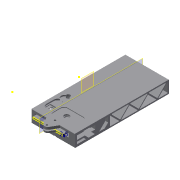
# Autodesk Inventor part: 01_SARS_detector_transmission_H20P_base_v0
Saved by Autodesk Inventor 2019.4 (Build 234330000, 330)
## iProperties
Created: 2020-10-16
Part Number: 01_SARS_detector_transmission_H20P_base_v0
Material: Generic
Document SubType Name: Modeling
Designer: diederichbenedict
Density: 1 g/cm^3
Appearance: Default
Author: diederichbenedict
Autodesk Inventor part; units mm, degrees
(part 1 of 2)
ref_plane "XZ Plane" through (0, 0, 0) normal (0, 1, 0) x (-1, 0, 0)
ref_plane "Work Plane1" through (47, 0, 0) normal (1, 0, 0) x (0, 1, 0)
sketch "Sketch1" plane through (47, 0, 0) normal (1, 0, 0) x (0, 1, 0)
  line L0 (-12.299, 54.1973) -> (-12.299, -85.8027) projected
  line L1 (-7.299, 21.1973) -> (-12.299, 21.1973)
  line L2 (-7.299, 17.1973) -> (-12.299, 17.1973)
  line L3 (-12.299, 21.6973) -> (-19.299, 21.6973)
  line L4 (-24.299, 26.6973) -> (-24.299, 42.4673)
  line L5 (-12.299, 51.1973) -> (-12.299, 56.0473) projected
  line L6 (-12.799, 51.1973) -> (-12.799, 56.0473) projected
  line L7 (-12.299, 54.1973) -> (-12.299, 57.6973) projected
  line L8 (-12.299, 56.3123) -> (-12.299, 70.3123)
  line L9 (-12.299, 56.3123) -> (-15.299, 56.3123)
  line L10 (-15.299, 56.3123) -> (-15.299, 21.6973)
  line L11 (-12.299, 16.6973) -> (-23.299, 16.6973)
  line L12 (-23.299, 16.6973) -> (-28.765, 22.1633)
  line L13 (-28.765, 22.1633) -> (-28.765, 48.2313)
  line L14 (-28.765, 48.2313) -> (-20.684, 56.3123)
  line L15 (-20.684, 56.3123) -> (-15.299, 56.3123)
  line L16 (-24.299, 42.4673) -> (-20.684, 46.0823)
  line L17 (-24.299, 42.4673) -> (-19.1866, 42.4673) construction
  line L18 (-20.684, 46.0823) -> (-15.299, 46.0823)
  line L19 (-19.299, 21.6973) -> (-24.299, 26.6973)
  line L20 (-12.999, 46.3323) -> (-17.739, 46.3323) projected
  line L21 (-17.739, 56.0623) -> (-12.999, 56.0623) projected
  line L22 (-12.299, 21.6973) -> (-12.299, 23.2191)
  line L23 (-15.299, 23.2191) -> (-12.299, 23.2191)
  line L24 (-12.299, 70.3123) -> (-32.299, 70.3123)
  line L25 (-32.299, 70.3123) -> (-32.299, -81.6877)
  line L26 (-32.299, -81.6877) -> (-12.299, -81.6877)
  line L27 (-12.299, -81.6877) -> (-12.299, 16.6973)
  line L28 (-12.299, -81.6877) -> (-32.299, -81.6877) construction
  line L29 (-32.299, -81.6877) -> (-32.299, 16.6973) construction
  line L30 (-32.299, 16.6973) -> (-12.299, 16.6973) construction
  line L31 (-12.299, 16.6973) -> (-12.299, -81.6877) construction
  line L32 (-14.299, -79.6877) -> (-30.299, -79.6877)
  line L33 (-30.299, -79.6877) -> (-30.299, 13.6973)
  line L34 (-30.299, 13.6973) -> (-14.299, 13.6973)
  line L35 (-14.299, 13.6973) -> (-14.299, -79.6877)
  line L36 (-12.299, 16.6973) -> (-15.299, 16.6973)
  line L37 (-15.299, 16.6973) -> (-15.299, 21.6973)
  line L38 (-15.299, 21.6973) -> (-12.299, 21.6973)
  line L39 (-12.299, 21.6973) -> (-12.299, 16.6973)
  line L40 (-12.299, 19.1973) -> (-25.799, 19.1973) construction
  line L41 (-25.799, 51.1973) -> (-12.799, 51.1973) construction
  line L42 (-25.799, 51.1973) -> (-25.799, 19.1973) construction
  line L43 (-28.6297, 52.6092) -> (-25.1023, 56.1367)
  line L44 (-25.1023, 56.1367) -> (-25.1023, 67.0836)
  line L45 (-25.1023, 67.0836) -> (-28.6297, 67.0836)
  line L46 (-28.6297, 67.0836) -> (-28.6297, 52.6092)
  point P0 (0, 0)
  point P1 (-24.299, 21.6973)
  dimension "d4" = 14
  dimension "d6" = 135
  dimension "d7" = 135
  dimension "d8" = 135
  dimension "d9" = 45
  dimension "d10" = 135
  dimension "d11" = 5
  dimension "d13" = 0.25
  dimension "d14" = 0.25
  dimension "d15" = 0.5
  dimension "d16" = 0.5
  dimension "d18" = 0
  dimension "d19" = 12
  dimension "d20" = 20
  dimension "d21" = 152
  dimension "d22" = 90
  dimension "d23" = 2
  dimension "d24" = 2
  dimension "d25" = 2
  dimension "d26" = 3
  dimension "d60" = 13.5
  dimension "d89" = 3
  constraints: 82 end point, 12 horizontal, 11 perpendicular, 9 point on line, 7 parallel, 4 vertical, 1 coincident, 1 collinear, 1 equal length, 1 midpoint, 9 other
  measures "d4" distance of L8.start L8.end
  measures "d6" angle of L11 L12
  measures "d7" angle of L12 L13
  measures "d8" angle of L13 L14
  measures "d9" angle of L17 L16
  measures "d10" angle of L18 L16
  measures "d11" distance of L3.end point (-24.299, 21.697)
  measures "d13" distance between parallel lines of L20 L18
  measures "d14" distance between parallel lines of L15 L21
  measures "d15" distance between parallel lines of L3 L1
  measures "d16" distance between parallel lines of L11 L2
  measures "d18" horizontal distance of L14.end L16.end
  measures "d20" distance of L8.end L24.end
  measures "d21" distance of L24.end L25.end
  measures "d22" angle of L25 L24
  measures "d24" distance between parallel lines of L26 L32
  measures "d25" distance between parallel lines of L29 L33
  measures "d26" distance between parallel lines of L30 L34
  measures "d60" distance of L40.end L40.start
  measures "d89" distance between parallel lines of L14 L43
extrude "Extrusion1" add sketch "Sketch1" along normal blind 50 and the other way blind 20 contours L0 L23 L10 L9 L7 L5 | L0 L3 L10 L23 | L9 L15 L14 L13 L12 L11 L0 L26 L25 L24 L8 L7 | L0 L11 L37 L3 | L10 L3 L19 L4 L16 L18
sketch "Sketch2" plane through (27, 0, 0) normal (-1, 0, 0) x (0, 0, 1)
  line L0 (13.6973, -30.299) -> (-79.6877, -30.299) projected
  line L1 (-79.6877, -30.299) -> (-79.6877, -14.299) projected
  line L2 (-79.6877, -14.299) -> (13.6973, -14.299) projected
  line L3 (13.6973, -14.299) -> (13.6973, -30.299) projected
  line L4 (70.3123, -12.299) -> (-81.6877, -12.299) projected
  line L5 (21.6973, -15.299) -> (21.6973, -19.299) projected
  line L6 (21.6973, -19.299) -> (26.6973, -24.299) projected
  line L7 (26.6973, -24.299) -> (42.4673, -24.299) projected
  line L8 (42.4673, -24.299) -> (46.0823, -20.684) projected
  line L9 (46.0823, -20.684) -> (46.0823, -15.299) projected
  line L10 (46.0823, -15.299) -> (56.3123, -15.299) projected
  line L11 (56.3123, -15.299) -> (56.3123, -20.684) projected
  line L12 (56.3123, -20.684) -> (48.2313, -28.765) projected
  line L13 (48.2313, -28.765) -> (22.1633, -28.765) projected
  line L14 (22.1633, -28.765) -> (16.6973, -23.299) projected
  line L15 (16.6973, -23.299) -> (16.6973, -15.299) projected
  line L16 (-81.6877, -12.299) -> (-81.6877, -32.299) projected
  line L17 (-81.6877, -32.299) -> (70.3123, -32.299) projected
  line L18 (70.3123, -32.299) -> (70.3123, -12.299) projected
  line L19 (-79.6877, -14.299) -> (-63.6877, -30.299)
  line L20 (-79.6877, -14.299) -> (-57.0603, -14.299) construction
  line L21 (-63.6877, -30.299) -> (-62.1877, -30.299)
  line L22 (-62.1877, -30.299) -> (-46.1877, -14.299)
  line L23 (-46.1877, -14.299) -> (-46.1877, -14.299)
  line L24 (-77.5664, -14.299) -> (-62.9377, -28.9277)
  line L25 (-62.9377, -28.9277) -> (-48.309, -14.299)
  line L26 (-79.6877, -14.299) -> (-77.5664, -14.299)
  line L27 (-48.309, -14.299) -> (-46.1877, -14.299)
  line L28 (16.6973, -15.299) -> (21.6973, -15.299) projected
  point P0 (0, 0)
  dimension "d31" = 45
  dimension "d_1" = 1.5
  dimension "d33" = 135
  dimension "d34" = 0
  dimension "d44" = 0.75
  dimension "d46" = 1.5
  constraints: 18 end point, 5 point on line, 2 collinear, 1 equal length, 1 horizontal, 1 parallel, 1 perpendicular
  measures "d31" angle of L19 L20
  measures "d_1" distance of L19.end L21.end
  measures "d33" angle of L22 L21
  measures "d34" distance of L22.end L23.end
  measures "d44" horizontal distance of L24.end L21.end
  measures "d46" distance between parallel lines of L22 L25
extrude "Extrusion2" add sketch "Sketch2" against normal up to surface (70 mm away) contours L0 L19 L2 L24 L25 L22
pattern_linear "Rectangular Pattern1" count 3 spacing 30 along (0, 0, 1) of "Extrusion2"
fillet "Fillet1" radius 0.75 20 edges at (62, -14.299, -79.6877) (62, -14.299, -77.5664) (62, -28.9277, -62.9377) (62, -30.299, -63.6877) (62, -30.299, -62.1877) (62, -16.049, -47.9377) (62, -16.049, -17.9377) (62, -28.9277, -32.9377) (62, -28.9277, -2.9377) (62, -30.299, 13.6973) (62, -30.299, -2.1877) (62, -30.299, -32.1877) (62, -30.299, -33.6877) (62, -30.299, -3.6877) (62, -14.299, 11.691) (62, -30.299, -79.6877) (62, -12.299, -81.6877) (62, -32.299, -81.6877) (62, -12.299, 70.3123) (62, -32.299, 70.3123)
sketch "Sketch3" plane through (27, -12.299, 69.5623) normal (0, 1, 0) x (1, 0, 0)
  line L0 (6.499, 14) -> (6.499, 22.73) projected
  arc A0 (6.999, 23.23) -> (6.499, 22.73) centre (6.999, 22.73) ccw projected
  arc A1 (6.499, 14) -> (6.999, 13.5) centre (6.999, 14) ccw projected
  line L1 (6.499, 14) -> (6.499, 22.73) projected
  line L2 (15.729, 13.5) -> (6.999, 13.5) projected
  arc A2 (15.729, 13.5) -> (16.229, 14) centre (15.729, 14) ccw projected
  line L3 (16.229, 22.73) -> (16.229, 14) projected
  arc A3 (16.229, 22.73) -> (15.729, 23.23) centre (15.729, 22.73) ccw projected
  line L4 (15.729, 23.23) -> (6.999, 23.23) projected
  line L5 (15.364, 14.75) -> (15.364, 22.75)
  line L6 (15.364, 22.75) -> (7.364, 22.75)
  line L7 (7.364, 22.75) -> (7.364, 14.75)
  line L8 (7.364, 14.75) -> (15.364, 14.75)
  circle A4 centre (11.364, 18.75) radius 4
  line L9 (0, -0.75) -> (70, -0.75) projected
  circle A5 centre (11.364, 47.25) radius 3
  point P0 (-27, 69.5623)
  dimension "d112" = 8
  dimension "d113" = 19.5
  dimension "d114" = 0
  dimension "d115" = 6
  dimension "d116" = 48
  constraints: 8 end point, 3 tangent, 2 centre point, 2 parallel, 1 perpendicular
  measures "d112" diameter of A4
  measures "d113" distance from line of A4.centre L9
  measures "d114" distance edge to line of A4 L6
  measures "d115" diameter of A5
  measures "d116" distance from line of L9 A5.centre
ref_plane "Work Plane2" through (7.664, -19.539, 38.4473) normal (0, -1, 0) x (1, 0, 0)
extrude "Extrusion3" cut sketch "Sketch3" against normal blind 10 contours L0 A0 L4 A3 L3 A2 L2 A1 | L8 A4 L5 | A4 L6 L5 | A4 | L8 L7 A4 | A4 L7 L6 | A5
sketch "Sketch4" plane through (27, 0, 0) normal (-1, 0, 0) x (0, 0, 1)
  line L0 (63.9473, -19.539) -> (38.4473, -19.539) construction
  line L1 (63.9473, -19.539) -> (63.9473, -18.239) construction
  line L2 (38.4473, -18.239) -> (63.9473, -18.239) construction
  line L3 (38.4473, -19.539) -> (38.4473, -18.239) construction
  line L4 (33.4473, -16.239) -> (71.8146, -16.239)
  line L5 (71.8146, -16.239) -> (71.8146, -22.539)
  line L6 (71.8146, -22.539) -> (33.4473, -22.539)
  line L7 (33.4473, -22.539) -> (33.4473, -16.239)
  point P0 (0, 0)
  dimension "d61" = 5
  dimension "d63" = 2
  dimension "d64" = 3
  constraints: 8 end point, 2 parallel, 1 horizontal, 1 perpendicular
  measures "d61" distance between parallel lines of L3 L7
  measures "d63" distance between parallel lines of L2 L4
  measures "d64" distance between parallel lines of L0 L6
extrude "Extrusion4" cut sketch "Sketch4" against normal blind 60
sketch "Sketch5" plane through (27, 0, 0) normal (-1, 0, 0) x (0, 0, 1)
  line L0 (33.4473, -16.239) -> (46.0823, -16.239) projected
  line L1 (46.0823, -16.239) -> (46.0823, -15.299) projected
  line L2 (46.0823, -15.299) -> (56.3123, -15.299) projected
  line L3 (56.3123, -15.299) -> (56.3123, -16.239) projected
  line L4 (56.3123, -16.239) -> (70.3123, -16.239) projected
  line L5 (70.3123, -22.539) -> (54.4573, -22.539) projected
  line L6 (54.4573, -22.539) -> (48.2313, -28.765) projected
  line L7 (48.2313, -28.765) -> (22.1633, -28.765) projected
  line L8 (22.1633, -28.765) -> (16.6973, -23.299) projected
  line L9 (16.6973, -23.299) -> (16.6973, -15.299) projected
  line L10 (16.6973, -15.299) -> (21.6973, -15.299) projected
  line L11 (21.6973, -15.299) -> (21.6973, -19.299) projected
  line L12 (21.6973, -19.299) -> (26.6973, -24.299) projected
  line L13 (26.6973, -24.299) -> (42.4673, -24.299) projected
  line L14 (42.4673, -24.299) -> (44.2273, -22.539) projected
  line L15 (44.2273, -22.539) -> (33.4473, -22.539) projected
  line L16 (33.4473, -22.539) -> (33.4473, -16.239) projected
  arc A0 (69.5623, -32.299) -> (70.3123, -31.549) centre (69.5623, -31.549) ccw projected
  line L17 (70.3123, -31.549) -> (70.3123, -22.539) projected
  arc A1 (70.3123, -13.049) -> (69.5623, -12.299) centre (69.5623, -13.049) ccw projected
  line L18 (69.5623, -12.299) -> (-80.9377, -12.299) projected
  arc A2 (-80.9377, -12.299) -> (-81.6877, -13.049) centre (-80.9377, -13.049) ccw projected
  line L19 (-81.6877, -13.049) -> (-81.6877, -31.549) projected
  arc A3 (-81.6877, -31.549) -> (-80.9377, -32.299) centre (-80.9377, -31.549) ccw projected
  line L20 (-80.9377, -32.299) -> (69.5623, -32.299) projected
  line L21 (13.6973, -14.414) -> (13.6973, -29.549) projected
  arc A4 (12.9473, -30.299) -> (13.6973, -29.549) centre (12.9473, -29.549) ccw projected
  line L22 (12.9473, -30.299) -> (-0.377, -30.299) projected
  line L23 (13.6973, -14.414) -> (-0.9074, -29.0187) projected
  line L24 (-4.968, -29.0187) -> (-17.4074, -16.5793) projected
  line L25 (-18.468, -16.5793) -> (-30.9074, -29.0187) projected
  line L26 (-2.4074, -28.3973) -> (10.4107, -15.5793) projected
  arc A5 (-3.468, -28.3973) -> (-2.4074, -28.3973) centre (-2.9377, -27.867) ccw projected
  line L27 (-16.877, -14.9883) -> (-3.468, -28.3973) projected
  line L28 (-16.1877, -14.299) -> (9.8803, -14.299) projected
  arc A6 (10.4107, -15.5793) -> (9.8803, -14.299) centre (9.8803, -15.049) ccw projected
  line L29 (-32.4074, -28.3973) -> (-18.9983, -14.9883) projected
  arc A7 (-33.468, -28.3973) -> (-32.4074, -28.3973) centre (-32.9377, -27.867) ccw projected
  line L30 (-46.877, -14.9883) -> (-33.468, -28.3973) projected
  line L31 (-46.1877, -14.299) -> (-19.6877, -14.299) projected
  line L32 (-34.968, -29.0187) -> (-47.4074, -16.5793) projected
  line L33 (-48.468, -16.5793) -> (-60.9074, -29.0187) projected
  line L34 (-62.4074, -28.3973) -> (-48.9983, -14.9883) projected
  arc A8 (-63.468, -28.3973) -> (-62.4074, -28.3973) centre (-62.9377, -27.867) ccw projected
  line L35 (-76.286, -15.5793) -> (-63.468, -28.3973) projected
  arc A9 (-75.7557, -14.299) -> (-76.286, -15.5793) centre (-75.7557, -15.049) ccw projected
  line L36 (-75.7557, -14.299) -> (-49.6877, -14.299) projected
  line L37 (-64.968, -29.0187) -> (-78.4074, -15.5793) projected
  arc A10 (-79.6877, -29.549) -> (-78.9377, -30.299) centre (-78.9377, -29.549) ccw projected
  line L38 (-79.6877, -29.549) -> (-79.6877, -16.1096) projected
  arc A11 (-78.4074, -15.5793) -> (-79.6877, -16.1096) centre (-78.9377, -16.1096) ccw projected
  line L39 (63.9473, -19.539) -> (38.4473, -19.539) projected
  line L40 (63.9473, -19.539) -> (63.9473, -18.239) projected
  line L41 (38.4473, -18.239) -> (63.9473, -18.239) projected
  line L42 (38.4473, -19.539) -> (38.4473, -18.239) projected
  line L43 (35.4473, -18.239) -> (35.4473, -19.439)
  line L44 (33.4473, -19.439) -> (33.4473, -18.239)
  line L45 (35.4473, -18.239) -> (37.4473, -18.239)
  line L46 (37.4473, -18.239) -> (37.4473, -20.739)
  line L47 (37.4473, -20.739) -> (35.4473, -20.739)
  line L48 (35.4473, -20.739) -> (35.4473, -18.239)
  line L49 (37.4473, -20.739) -> (64.4473, -20.739)
  line L50 (64.4473, -20.739) -> (64.4473, -19.739)
  line L51 (64.4473, -19.739) -> (37.4473, -19.739)
  line L52 (37.4473, -19.739) -> (37.4473, -20.739)
  line L53 (64.4473, -20.739) -> (74.4473, -20.739)
  line L54 (74.4473, -20.739) -> (74.4473, -18.239)
  line L55 (74.4473, -18.239) -> (64.4473, -18.239)
  line L56 (64.4473, -18.239) -> (64.4473, -20.739)
  line L57 (70.3123, -16.239) -> (70.3123, -13.049) projected
  line L58 (67.0836, -25.1023) -> (67.0836, -28.6297) projected
  line L59 (67.0836, -28.6297) -> (52.6092, -28.6297) projected
  line L60 (52.6092, -28.6297) -> (56.1367, -25.1023) projected
  line L61 (56.1367, -25.1023) -> (67.0836, -25.1023) projected
  arc A12 (-17.4074, -16.5793) -> (-18.468, -16.5793) centre (-17.9377, -17.1096) ccw projected
  arc A13 (-47.4074, -16.5793) -> (-48.468, -16.5793) centre (-47.9377, -17.1096) ccw projected
  line L62 (-5.4983, -30.299) -> (-30.377, -30.299) projected
  arc A14 (-30.9074, -29.0187) -> (-30.377, -30.299) centre (-30.377, -29.549) ccw projected
  arc A15 (-5.4983, -30.299) -> (-4.968, -29.0187) centre (-5.4983, -29.549) ccw projected
  arc A16 (-0.9074, -29.0187) -> (-0.377, -30.299) centre (-0.377, -29.549) ccw projected
  line L63 (-16.1877, -14.299) -> (-16.877, -14.9883) projected
  line L64 (-18.9983, -14.9883) -> (-19.6877, -14.299) projected
  line L65 (-46.1877, -14.299) -> (-46.877, -14.9883) projected
  line L66 (-48.9983, -14.9883) -> (-49.6877, -14.299) projected
  line L67 (-35.4983, -30.299) -> (-60.377, -30.299) projected
  arc A17 (-60.9074, -29.0187) -> (-60.377, -30.299) centre (-60.377, -29.549) ccw projected
  arc A18 (-35.4983, -30.299) -> (-34.968, -29.0187) centre (-35.4983, -29.549) ccw projected
  line L68 (-65.4983, -30.299) -> (-78.9377, -30.299) projected
  arc A19 (-65.4983, -30.299) -> (-64.968, -29.0187) centre (-65.4983, -29.549) ccw projected
  line L69 (35.4473, -20.739) -> (33.4473, -20.739)
  line L70 (33.4473, -20.739) -> (33.4473, -19.739)
  line L71 (33.4473, -19.739) -> (35.4473, -19.739)
  line L72 (35.4473, -19.739) -> (35.4473, -20.739)
  point P0 (0, 0)
  dimension "d67" = 2
  dimension "d68" = 1.2
  dimension "d69" = 2
  dimension "d70" = 2.5
  dimension "d71" = 1
  dimension "d72" = 27
  dimension "d73" = 10
  dimension "d98" = 0
  constraints: 36 end point, 9 parallel, 4 horizontal, 4 perpendicular, 2 point on line
  measures "d67" distance of L43.end L44.start
  measures "d68" distance of L43.start L43.end
  measures "d69" distance of L46.end L47.end
  measures "d70" distance of L45.end L46.end
  measures "d71" distance of L50.end L49.end
  measures "d72" distance between parallel lines of L50 L46
  measures "d73" distance of L55.end L54.end
  measures "d98" distance between parallel lines of L45 L41
extrude "Extrusion5" add sketch "Sketch5" against normal blind 55 contours L71 L48 L69 L16 | L48 L43 L45 L46 L47 | L46 L51 L50 L49 | L50 L56 L55 L54 L53
sketch "Sketch6" plane through (27, -12.299, 69.5623) normal (0, 1, 0) x (1, 0, 0)
  circle A0 centre (11.364, 50.365) radius 2 projected
  arc A1 (16.214, 29.865) -> (6.514, 29.865) centre (11.364, 29.865) ccw projected
  line L0 (6.514, 29.865) -> (6.514, 18.365) projected
  arc A2 (6.514, 18.365) -> (16.214, 18.365) centre (11.364, 18.365) ccw projected
  line L1 (16.214, 18.365) -> (16.214, 29.865) projected
  circle A3 centre (11.364, 41.365) radius 4.315 projected
  arc A4 (6.364, 158.865) -> (2.864, 155.365) centre (6.364, 155.365) ccw projected
  line L2 (65.244, 158.865) -> (6.364, 158.865) projected
  arc A5 (68.744, 155.365) -> (65.244, 158.865) centre (65.244, 155.365) ccw projected
  line L3 (68.744, 15.365) -> (68.744, 155.365) projected
  arc A6 (65.244, 11.865) -> (68.744, 15.365) centre (65.244, 15.365) ccw projected
  line L4 (6.364, 11.865) -> (65.244, 11.865) projected
  arc A7 (2.864, 15.365) -> (6.364, 11.865) centre (6.364, 15.365) ccw projected
  line L5 (2.864, 155.365) -> (2.864, 15.365) projected
  arc A8 (17.714, 29.865) -> (5.014, 29.865) centre (11.364, 29.865) ccw
  line L6 (5.014, 29.865) -> (5.014, 18.365)
  arc A9 (5.014, 18.365) -> (17.714, 18.365) centre (11.364, 18.365) ccw
  line L7 (17.714, 18.365) -> (17.714, 29.865)
  circle A10 centre (11.364, 41.365) radius 5.815
  point P0 (-27, 69.5623)
  dimension "d76" = 1.5
  dimension "d77" = 1.5
  constraints: 4 end point, 4 point on circle, 3 centre point, 3 other
  measures "d76" distance between parallel lines of L1 L7
  measures "d77" radial gap between concentric circles of A3 A10
extrude "Extrusion6" cut sketch "Sketch6" against normal blind 2 contours L1 A2 L0 A1 | A3 | L7 A9 L6 A8 A10 | A10 A8 | A8 A10
sketch "Sketch7" plane through (27, 0, 0) normal (-1, 0, 0) x (0, 0, 1)
  line L0 (70.3123, -22.539) -> (54.4573, -22.539) projected
  line L1 (54.4573, -22.539) -> (48.2313, -28.765) projected
  line L2 (48.2313, -28.765) -> (22.1633, -28.765) projected
  line L3 (22.1633, -28.765) -> (16.6973, -23.299) projected
  line L4 (16.6973, -23.299) -> (16.6973, -15.299) projected
  line L5 (16.6973, -15.299) -> (21.6973, -15.299) projected
  line L6 (21.6973, -15.299) -> (21.6973, -19.299) projected
  line L7 (21.6973, -19.299) -> (26.6973, -24.299) projected
  line L8 (26.6973, -24.299) -> (42.4673, -24.299) projected
  line L9 (42.4673, -24.299) -> (44.2273, -22.539) projected
  line L10 (44.2273, -22.539) -> (33.4473, -22.539) projected
  line L11 (33.4473, -22.539) -> (33.4473, -20.739) projected
  line L12 (33.4473, -16.239) -> (46.0823, -16.239) projected
  line L13 (46.0823, -16.239) -> (46.0823, -15.299) projected
  line L14 (46.0823, -15.299) -> (56.3123, -15.299) projected
  line L15 (56.3123, -15.299) -> (56.3123, -16.239) projected
  line L16 (56.3123, -16.239) -> (70.3123, -16.239) projected
  line L17 (70.3123, -16.239) -> (70.3123, -13.049) projected
  arc A0 (70.3123, -13.049) -> (69.5623, -12.299) centre (69.5623, -13.049) ccw projected
  line L18 (69.5623, -12.299) -> (-80.9377, -12.299) projected
  arc A1 (-80.9377, -12.299) -> (-81.6877, -13.049) centre (-80.9377, -13.049) ccw projected
  line L19 (-81.6877, -13.049) -> (-81.6877, -31.549) projected
  arc A2 (-81.6877, -31.549) -> (-80.9377, -32.299) centre (-80.9377, -31.549) ccw projected
  line L20 (-80.9377, -32.299) -> (69.5623, -32.299) projected
  arc A3 (69.5623, -32.299) -> (70.3123, -31.549) centre (69.5623, -31.549) ccw projected
  line L21 (70.3123, -31.549) -> (70.3123, -22.539) projected
  line L22 (-64.968, -29.0187) -> (-78.4074, -15.5793) projected
  line L23 (-65.4983, -30.299) -> (-78.9377, -30.299) projected
  arc A4 (-79.6877, -29.549) -> (-78.9377, -30.299) centre (-78.9377, -29.549) ccw projected
  line L24 (-79.6877, -29.549) -> (-79.6877, -16.1096) projected
  arc A5 (-78.4074, -15.5793) -> (-79.6877, -16.1096) centre (-78.9377, -16.1096) ccw projected
  line L25 (-62.4074, -28.3973) -> (-48.9983, -14.9883) projected
  arc A6 (-63.468, -28.3973) -> (-62.4074, -28.3973) centre (-62.9377, -27.867) ccw projected
  line L26 (-76.286, -15.5793) -> (-63.468, -28.3973) projected
  arc A7 (-75.7557, -14.299) -> (-76.286, -15.5793) centre (-75.7557, -15.049) ccw projected
  line L27 (-75.7557, -14.299) -> (-49.6877, -14.299) projected
  line L28 (-34.968, -29.0187) -> (-47.4074, -16.5793) projected
  line L29 (-48.468, -16.5793) -> (-60.9074, -29.0187) projected
  line L30 (-32.4074, -28.3973) -> (-18.9983, -14.9883) projected
  arc A8 (-33.468, -28.3973) -> (-32.4074, -28.3973) centre (-32.9377, -27.867) ccw projected
  line L31 (-46.877, -14.9883) -> (-33.468, -28.3973) projected
  line L32 (-46.1877, -14.299) -> (-19.6877, -14.299) projected
  line L33 (-2.4074, -28.3973) -> (10.4107, -15.5793) projected
  arc A9 (-3.468, -28.3973) -> (-2.4074, -28.3973) centre (-2.9377, -27.867) ccw projected
  line L34 (-16.877, -14.9883) -> (-3.468, -28.3973) projected
  line L35 (-16.1877, -14.299) -> (9.8803, -14.299) projected
  arc A10 (10.4107, -15.5793) -> (9.8803, -14.299) centre (9.8803, -15.049) ccw projected
  line L36 (-4.968, -29.0187) -> (-17.4074, -16.5793) projected
  line L37 (-18.468, -16.5793) -> (-30.9074, -29.0187) projected
  line L38 (13.6973, -14.414) -> (13.6973, -29.549) projected
  arc A11 (12.9473, -30.299) -> (13.6973, -29.549) centre (12.9473, -29.549) ccw projected
  line L39 (13.6973, -14.414) -> (-0.9074, -29.0187) projected
  line L40 (70.9625, -17.239) -> (33.4473, -17.239)
  line L41 (33.4473, -17.239) -> (33.4473, -22.539)
  line L42 (33.4473, -22.539) -> (70.9625, -22.539)
  line L43 (70.9625, -22.539) -> (70.9625, -17.239)
  line L44 (70.3123, -31.549) -> (70.3123, -22.539) projected
  line L45 (70.3123, -22.539) -> (77.4578, -22.539)
  line L46 (77.4578, -22.539) -> (77.4578, -17.239)
  line L47 (77.4578, -17.239) -> (70.3123, -17.239)
  line L48 (70.3123, -17.239) -> (70.3123, -22.539)
  line L49 (67.0836, -25.1023) -> (67.0836, -28.6297) projected
  line L50 (67.0836, -28.6297) -> (52.6092, -28.6297) projected
  line L51 (52.6092, -28.6297) -> (56.1367, -25.1023) projected
  line L52 (56.1367, -25.1023) -> (67.0836, -25.1023) projected
  arc A12 (-17.4074, -16.5793) -> (-18.468, -16.5793) centre (-17.9377, -17.1096) ccw projected
  arc A13 (-47.4074, -16.5793) -> (-48.468, -16.5793) centre (-47.9377, -17.1096) ccw projected
  line L53 (-5.4983, -30.299) -> (-30.377, -30.299) projected
  arc A14 (-30.9074, -29.0187) -> (-30.377, -30.299) centre (-30.377, -29.549) ccw projected
  arc A15 (-5.4983, -30.299) -> (-4.968, -29.0187) centre (-5.4983, -29.549) ccw projected
  line L54 (12.9473, -30.299) -> (-0.377, -30.299) projected
  arc A16 (-0.9074, -29.0187) -> (-0.377, -30.299) centre (-0.377, -29.549) ccw projected
  line L55 (-16.1877, -14.299) -> (-16.877, -14.9883) projected
  line L56 (-18.9983, -14.9883) -> (-19.6877, -14.299) projected
  line L57 (-46.1877, -14.299) -> (-46.877, -14.9883) projected
  line L58 (-48.9983, -14.9883) -> (-49.6877, -14.299) projected
  line L59 (-35.4983, -30.299) -> (-60.377, -30.299) projected
  arc A17 (-60.9074, -29.0187) -> (-60.377, -30.299) centre (-60.377, -29.549) ccw projected
  arc A18 (-35.4983, -30.299) -> (-34.968, -29.0187) centre (-35.4983, -29.549) ccw projected
  arc A19 (-65.4983, -30.299) -> (-64.968, -29.0187) centre (-65.4983, -29.549) ccw projected
  line L60 (33.4473, -20.739) -> (74.4473, -20.739) projected
  line L61 (74.4473, -20.739) -> (74.4473, -18.239) projected
  line L62 (74.4473, -18.239) -> (64.4473, -18.239) projected
  line L63 (64.4473, -18.239) -> (64.4473, -19.739) projected
  line L64 (37.4473, -19.739) -> (64.4473, -19.739) projected
  line L65 (37.4473, -18.239) -> (37.4473, -19.739) projected
  line L66 (35.4473, -18.239) -> (37.4473, -18.239) projected
  line L67 (35.4473, -19.739) -> (35.4473, -18.239) projected
  line L68 (33.4473, -19.739) -> (35.4473, -19.739) projected
  line L69 (33.4473, -19.739) -> (33.4473, -16.239) projected
  point P0 (0, 0)
  constraints: 16 end point, 4 parallel, 2 horizontal, 2 perpendicular, 1 other
extrude "Extrusion7" cut sketch "Sketch7" against normal blind 6 contours L48 L60 L43 L42 | L0 L42 L10 L11 L60 L48 | L43 L60 L61 L62 L47 L46 L45 | L60 L41 L68 L67 L66 L65 L64 L63 L62 L48 | L48 L62 L43 L60 | L43 L62 L61 L60 | L62 L63 L64 L65 L66 L67 L68 L41 L40 L48 | L48 L40 L43 L62
sketch "Sketch8" plane through (27, 0, 0) normal (-1, 0, 0) x (0, 0, 1)
  line L0 (33.4473, -22.539) -> (33.4473, -16.239) projected
  line L1 (33.4473, -16.239) -> (46.0823, -16.239) projected
  line L2 (46.0823, -16.239) -> (46.0823, -15.299) projected
  line L3 (46.0823, -15.299) -> (56.3123, -15.299) projected
  line L4 (56.3123, -15.299) -> (56.3123, -16.239) projected
  line L5 (56.3123, -16.239) -> (70.3123, -16.239) projected
  line L6 (70.3123, -16.239) -> (70.3123, -13.049) projected
  arc A0 (70.3123, -13.049) -> (69.5623, -12.299) centre (69.5623, -13.049) ccw projected
  line L7 (69.5623, -12.299) -> (-80.9377, -12.299) projected
  arc A1 (-80.9377, -12.299) -> (-81.6877, -13.049) centre (-80.9377, -13.049) ccw projected
  line L8 (-81.6877, -13.049) -> (-81.6877, -31.549) projected
  arc A2 (-81.6877, -31.549) -> (-80.9377, -32.299) centre (-80.9377, -31.549) ccw projected
  line L9 (-80.9377, -32.299) -> (69.5623, -32.299) projected
  arc A3 (69.5623, -32.299) -> (70.3123, -31.549) centre (69.5623, -31.549) ccw projected
  line L10 (70.3123, -31.549) -> (70.3123, -22.539) projected
  line L11 (70.3123, -22.539) -> (54.4573, -22.539) projected
  line L12 (54.4573, -22.539) -> (48.2313, -28.765) projected
  line L13 (48.2313, -28.765) -> (22.1633, -28.765) projected
  line L14 (22.1633, -28.765) -> (16.6973, -23.299) projected
  line L15 (16.6973, -23.299) -> (16.6973, -15.299) projected
  line L16 (16.6973, -15.299) -> (21.6973, -15.299) projected
  line L17 (21.6973, -15.299) -> (21.6973, -19.299) projected
  line L18 (21.6973, -19.299) -> (26.6973, -24.299) projected
  line L19 (26.6973, -24.299) -> (42.4673, -24.299) projected
  line L20 (42.4673, -24.299) -> (44.2273, -22.539) projected
  line L21 (44.2273, -22.539) -> (33.4473, -22.539) projected
  line L22 (-64.968, -29.0187) -> (-78.4074, -15.5793) projected
  line L23 (-65.4983, -30.299) -> (-78.9377, -30.299) projected
  arc A4 (-79.6877, -29.549) -> (-78.9377, -30.299) centre (-78.9377, -29.549) ccw projected
  line L24 (-79.6877, -29.549) -> (-79.6877, -16.1096) projected
  arc A5 (-78.4074, -15.5793) -> (-79.6877, -16.1096) centre (-78.9377, -16.1096) ccw projected
  line L25 (-62.4074, -28.3973) -> (-48.9983, -14.9883) projected
  arc A6 (-63.468, -28.3973) -> (-62.4074, -28.3973) centre (-62.9377, -27.867) ccw projected
  line L26 (-76.286, -15.5793) -> (-63.468, -28.3973) projected
  arc A7 (-75.7557, -14.299) -> (-76.286, -15.5793) centre (-75.7557, -15.049) ccw projected
  line L27 (-75.7557, -14.299) -> (-49.6877, -14.299) projected
  line L28 (-34.968, -29.0187) -> (-47.4074, -16.5793) projected
  line L29 (-48.468, -16.5793) -> (-60.9074, -29.0187) projected
  line L30 (-32.4074, -28.3973) -> (-18.9983, -14.9883) projected
  arc A8 (-33.468, -28.3973) -> (-32.4074, -28.3973) centre (-32.9377, -27.867) ccw projected
  line L31 (-46.877, -14.9883) -> (-33.468, -28.3973) projected
  line L32 (-46.1877, -14.299) -> (-19.6877, -14.299) projected
  line L33 (-2.4074, -28.3973) -> (10.4107, -15.5793) projected
  arc A9 (-3.468, -28.3973) -> (-2.4074, -28.3973) centre (-2.9377, -27.867) ccw projected
  line L34 (-16.877, -14.9883) -> (-3.468, -28.3973) projected
  line L35 (-16.1877, -14.299) -> (9.8803, -14.299) projected
  arc A10 (10.4107, -15.5793) -> (9.8803, -14.299) centre (9.8803, -15.049) ccw projected
  line L36 (-4.968, -29.0187) -> (-17.4074, -16.5793) projected
  line L37 (-18.468, -16.5793) -> (-30.9074, -29.0187) projected
  line L38 (13.6973, -14.414) -> (13.6973, -29.549) projected
  arc A11 (12.9473, -30.299) -> (13.6973, -29.549) centre (12.9473, -29.549) ccw projected
  line L39 (13.6973, -14.414) -> (-0.9074, -29.0187) projected
  line L40 (56.3123, -16.239) -> (70.3123, -16.239) projected
  line L41 (70.3123, -22.539) -> (54.4573, -22.539) projected
  line L42 (70.3123, -16.239) -> (67.3123, -16.239)
  line L43 (67.3123, -16.239) -> (67.3123, -22.539)
  line L44 (67.3123, -22.539) -> (70.3123, -22.539)
  line L45 (70.3123, -22.539) -> (70.3123, -16.239)
  line L46 (67.0836, -25.1023) -> (67.0836, -28.6297) projected
  line L47 (67.0836, -28.6297) -> (52.6092, -28.6297) projected
  line L48 (52.6092, -28.6297) -> (56.1367, -25.1023) projected
  line L49 (56.1367, -25.1023) -> (67.0836, -25.1023) projected
  arc A12 (-47.4074, -16.5793) -> (-48.468, -16.5793) centre (-47.9377, -17.1096) ccw projected
  arc A13 (-17.4074, -16.5793) -> (-18.468, -16.5793) centre (-17.9377, -17.1096) ccw projected
  arc A14 (-65.4983, -30.299) -> (-64.968, -29.0187) centre (-65.4983, -29.549) ccw projected
  line L50 (-35.4983, -30.299) -> (-60.377, -30.299) projected
  arc A15 (-60.9074, -29.0187) -> (-60.377, -30.299) centre (-60.377, -29.549) ccw projected
  arc A16 (-35.4983, -30.299) -> (-34.968, -29.0187) centre (-35.4983, -29.549) ccw projected
  line L51 (-48.9983, -14.9883) -> (-49.6877, -14.299) projected
  line L52 (-18.9983, -14.9883) -> (-19.6877, -14.299) projected
  line L53 (-46.1877, -14.299) -> (-46.877, -14.9883) projected
  line L54 (-16.1877, -14.299) -> (-16.877, -14.9883) projected
  line L55 (12.9473, -30.299) -> (-0.377, -30.299) projected
  arc A17 (-0.9074, -29.0187) -> (-0.377, -30.299) centre (-0.377, -29.549) ccw projected
  line L56 (-5.4983, -30.299) -> (-30.377, -30.299) projected
  arc A18 (-30.9074, -29.0187) -> (-30.377, -30.299) centre (-30.377, -29.549) ccw projected
  arc A19 (-5.4983, -30.299) -> (-4.968, -29.0187) centre (-5.4983, -29.549) ccw projected
  point P0 (0, 0)
  dimension "d83" = 3
  constraints: 8 end point, 2 parallel, 1 horizontal, 1 perpendicular, 1 point on line
  measures "d83" distance of L44.end L43.end
extrude "Extrusion8" add sketch "Sketch8" against normal blind 5 contours L5 L45 L11 L43
ref_plane "Work Plane3" through (47, 0, 0) normal (-1, 0, 0) x (0, 0, 1)
sketch "Sketch9" plane through (47, 0, 0) normal (-1, 0, 0) x (0, 0, 1)
  line L0 (-49.6877, -14.299) -> (-75.7557, -14.299) projected
  line L1 (-3.468, -28.3973) -> (-16.877, -14.9883) projected
  arc A0 (-3.468, -28.3973) -> (-2.4074, -28.3973) centre (-2.9377, -27.867) ccw projected
  line L2 (10.4107, -15.5793) -> (-2.4074, -28.3973) projected
  arc A1 (10.4107, -15.5793) -> (9.8803, -14.299) centre (9.8803, -15.049) ccw projected
  line L3 (-19.6877, -14.299) -> (-46.1877, -14.299) projected
  line L4 (-33.468, -28.3973) -> (-46.877, -14.9883) projected
  arc A2 (-33.468, -28.3973) -> (-32.4074, -28.3973) centre (-32.9377, -27.867) ccw projected
  line L5 (-18.9983, -14.9883) -> (-32.4074, -28.3973) projected
  line L6 (-30.377, -30.299) -> (-5.4983, -30.299) projected
  line L7 (-17.4074, -16.5793) -> (-4.968, -29.0187) projected
  line L8 (-30.9074, -29.0187) -> (-18.468, -16.5793) projected
  line L9 (-47.4074, -16.5793) -> (-34.968, -29.0187) projected
  line L10 (-60.9074, -29.0187) -> (-48.468, -16.5793) projected
  arc A3 (69.5623, -32.299) -> (70.3123, -31.549) centre (69.5623, -31.549) ccw projected
  line L11 (69.5623, -32.299) -> (-80.9377, -32.299) projected
  arc A4 (-81.6877, -31.549) -> (-80.9377, -32.299) centre (-80.9377, -31.549) ccw projected
  line L12 (-81.6877, -31.549) -> (-81.6877, -13.049) projected
  arc A5 (-80.9377, -12.299) -> (-81.6877, -13.049) centre (-80.9377, -13.049) ccw projected
  line L13 (-80.9377, -12.299) -> (69.5623, -12.299) projected
  arc A6 (70.3123, -13.049) -> (69.5623, -12.299) centre (69.5623, -13.049) ccw construction
  line L14 (70.3123, -13.049) -> (70.3123, -31.549) projected
  line L15 (16.6973, -15.299) -> (16.6973, -23.299) projected
  line L16 (16.6973, -23.299) -> (22.1633, -28.765) projected
  line L17 (22.1633, -28.765) -> (48.2313, -28.765) projected
  line L18 (48.2313, -28.765) -> (56.3123, -20.684) projected
  line L19 (56.3123, -20.684) -> (56.3123, -15.299) projected
  line L20 (56.3123, -15.299) -> (46.0823, -15.299) construction
  line L21 (46.0823, -15.299) -> (46.0823, -20.684) projected
  line L22 (46.0823, -20.684) -> (42.4673, -24.299) projected
  line L23 (42.4673, -24.299) -> (26.6973, -24.299) projected
  line L24 (26.6973, -24.299) -> (21.6973, -19.299) projected
  line L25 (21.6973, -19.299) -> (21.6973, -15.299) projected
  line L26 (21.6973, -15.299) -> (16.6973, -15.299) projected
  line L27 (52.6092, -28.6297) -> (67.0836, -28.6297) projected
  line L28 (67.0836, -28.6297) -> (67.0836, -25.1023) projected
  line L29 (67.0836, -25.1023) -> (56.1367, -25.1023) projected
  line L30 (56.1367, -25.1023) -> (52.6092, -28.6297) projected
  arc A7 (12.9473, -30.299) -> (13.6973, -29.549) centre (12.9473, -29.549) ccw projected
  line L31 (13.6973, -29.549) -> (13.6973, -14.414) projected
  line L32 (-0.9074, -29.0187) -> (13.6973, -14.414) projected
  line L33 (-79.6877, -16.1096) -> (-79.6877, -29.549) projected
  arc A8 (-79.6877, -29.549) -> (-78.9377, -30.299) centre (-78.9377, -29.549) ccw projected
  line L34 (-78.4074, -15.5793) -> (-64.968, -29.0187) projected
  arc A9 (-78.4074, -15.5793) -> (-79.6877, -16.1096) centre (-78.9377, -16.1096) ccw projected
  line L35 (9.8803, -14.299) -> (-16.1877, -14.299) projected
  arc A10 (-75.7557, -14.299) -> (-76.286, -15.5793) centre (-75.7557, -15.049) ccw projected
  line L36 (-63.468, -28.3973) -> (-76.286, -15.5793) projected
  arc A11 (-63.468, -28.3973) -> (-62.4074, -28.3973) centre (-62.9377, -27.867) ccw projected
  line L37 (-48.9983, -14.9883) -> (-62.4074, -28.3973) projected
  line L38 (67.3123, -22.539) -> (54.4573, -22.539) projected
  line L39 (54.4573, -22.539) -> (48.2313, -28.765) projected
  line L40 (48.2313, -28.765) -> (22.1633, -28.765) projected
  line L41 (22.1633, -28.765) -> (16.6973, -23.299) projected
  line L42 (16.6973, -23.299) -> (16.6973, -15.299) projected
  line L43 (16.6973, -15.299) -> (21.6973, -15.299) projected
  line L44 (21.6973, -15.299) -> (21.6973, -19.299) projected
  line L45 (21.6973, -19.299) -> (26.6973, -24.299) projected
  line L46 (26.6973, -24.299) -> (42.4673, -24.299) projected
  line L47 (42.4673, -24.299) -> (44.2273, -22.539) projected
  line L48 (44.2273, -22.539) -> (33.4473, -22.539) projected
  line L49 (33.4473, -22.539) -> (33.4473, -16.239) projected
  line L50 (33.4473, -16.239) -> (46.0823, -16.239) construction
  line L51 (46.0823, -16.239) -> (46.0823, -15.299) construction
  line L52 (46.0823, -15.299) -> (56.3123, -15.299) construction
  line L53 (56.3123, -15.299) -> (56.3123, -16.239) construction
  line L54 (56.3123, -16.239) -> (67.3123, -16.239) construction
  line L55 (67.3123, -22.539) -> (67.3123, -16.239) projected
  line L56 (70.3123, -31.549) -> (70.3123, -13.049) projected
  arc A12 (70.3123, -13.049) -> (69.5623, -12.299) centre (69.5623, -13.049) ccw construction
  line L57 (69.5623, -12.299) -> (-80.9377, -12.299) projected
  arc A13 (-80.9377, -12.299) -> (-81.6877, -13.049) centre (-80.9377, -13.049) ccw projected
  line L58 (-81.6877, -13.049) -> (-81.6877, -31.549) projected
  arc A14 (-81.6877, -31.549) -> (-80.9377, -32.299) centre (-80.9377, -31.549) ccw projected
  line L59 (-80.9377, -32.299) -> (69.5623, -32.299) projected
  arc A15 (69.5623, -32.299) -> (70.3123, -31.549) centre (69.5623, -31.549) ccw projected
  line L60 (13.6973, -14.414) -> (13.6973, -29.549) projected
  arc A16 (12.9473, -30.299) -> (13.6973, -29.549) centre (12.9473, -29.549) ccw projected
  line L61 (12.9473, -30.299) -> (-0.377, -30.299) projected
  line L62 (13.6973, -14.414) -> (-0.9074, -29.0187) projected
  line L63 (-4.968, -29.0187) -> (-17.4074, -16.5793) projected
  line L64 (-18.468, -16.5793) -> (-30.9074, -29.0187) projected
  line L65 (-2.4074, -28.3973) -> (10.4107, -15.5793) projected
  arc A17 (-3.468, -28.3973) -> (-2.4074, -28.3973) centre (-2.9377, -27.867) ccw projected
  line L66 (-16.877, -14.9883) -> (-3.468, -28.3973) projected
  line L67 (-46.1877, -14.299) -> (-19.6877, -14.299) projected
  arc A18 (10.4107, -15.5793) -> (9.8803, -14.299) centre (9.8803, -15.049) ccw projected
  line L68 (-32.4074, -28.3973) -> (-18.9983, -14.9883) projected
  arc A19 (-33.468, -28.3973) -> (-32.4074, -28.3973) centre (-32.9377, -27.867) ccw projected
  line L69 (-46.877, -14.9883) -> (-33.468, -28.3973) projected
  line L70 (-16.1877, -14.299) -> (9.8803, -14.299) projected
  line L71 (-34.968, -29.0187) -> (-47.4074, -16.5793) projected
  line L72 (-48.468, -16.5793) -> (-60.9074, -29.0187) projected
  line L73 (-62.4074, -28.3973) -> (-48.9983, -14.9883) projected
  arc A20 (-63.468, -28.3973) -> (-62.4074, -28.3973) centre (-62.9377, -27.867) ccw projected
  line L74 (-76.286, -15.5793) -> (-63.468, -28.3973) projected
  arc A21 (-75.7557, -14.299) -> (-76.286, -15.5793) centre (-75.7557, -15.049) ccw projected
  line L75 (-75.7557, -14.299) -> (-49.6877, -14.299) projected
  line L76 (-64.968, -29.0187) -> (-78.4074, -15.5793) projected
  arc A22 (-79.6877, -29.549) -> (-78.9377, -30.299) centre (-78.9377, -29.549) ccw projected
  line L77 (-79.6877, -29.549) -> (-79.6877, -16.1096) projected
  arc A23 (-78.4074, -15.5793) -> (-79.6877, -16.1096) centre (-78.9377, -16.1096) ccw projected
  line L78 (67.0836, -28.6297) -> (52.6092, -28.6297) projected
  line L79 (52.6092, -28.6297) -> (56.1367, -25.1023) projected
  line L80 (56.1367, -25.1023) -> (67.0836, -25.1023) projected
  line L81 (67.0836, -25.1023) -> (67.0836, -28.6297) projected
  line L82 (44.2273, -22.539) -> (54.4573, -22.539)
  line L83 (54.4573, -22.539) -> (48.2313, -28.765) projected
  arc A24 (-47.4074, -16.5793) -> (-48.468, -16.5793) centre (-47.9377, -17.1096) ccw projected
  arc A25 (-17.4074, -16.5793) -> (-18.468, -16.5793) centre (-17.9377, -17.1096) ccw projected
  arc A26 (-17.4074, -16.5793) -> (-18.468, -16.5793) centre (-17.9377, -17.1096) ccw projected
  arc A27 (-47.4074, -16.5793) -> (-48.468, -16.5793) centre (-47.9377, -17.1096) ccw projected
  line L84 (-65.4983, -30.299) -> (-78.9377, -30.299) projected
  arc A28 (-65.4983, -30.299) -> (-64.968, -29.0187) centre (-65.4983, -29.549) ccw projected
  line L85 (-35.4983, -30.299) -> (-60.377, -30.299) projected
  arc A29 (-60.9074, -29.0187) -> (-60.377, -30.299) centre (-60.377, -29.549) ccw projected
  arc A30 (-35.4983, -30.299) -> (-34.968, -29.0187) centre (-35.4983, -29.549) ccw projected
  line L86 (-48.9983, -14.9883) -> (-49.6877, -14.299) projected
  line L87 (-18.9983, -14.9883) -> (-19.6877, -14.299) projected
  line L88 (-46.1877, -14.299) -> (-46.877, -14.9883) projected
  line L89 (-16.1877, -14.299) -> (-16.877, -14.9883) projected
  arc A31 (-0.9074, -29.0187) -> (-0.377, -30.299) centre (-0.377, -29.549) ccw projected
  line L90 (-5.4983, -30.299) -> (-30.377, -30.299) projected
  arc A32 (-30.9074, -29.0187) -> (-30.377, -30.299) centre (-30.377, -29.549) ccw projected
  arc A33 (-5.4983, -30.299) -> (-4.968, -29.0187) centre (-5.4983, -29.549) ccw projected
  line L91 (-0.377, -30.299) -> (12.9473, -30.299) projected
  arc A34 (-0.9074, -29.0187) -> (-0.377, -30.299) centre (-0.377, -29.549) ccw projected
  line L92 (-16.877, -14.9883) -> (-16.1877, -14.299) projected
  line L93 (-46.877, -14.9883) -> (-46.1877, -14.299) projected
  line L94 (-19.6877, -14.299) -> (-18.9983, -14.9883) projected
  line L95 (-60.377, -30.299) -> (-35.4983, -30.299) projected
  arc A35 (-35.4983, -30.299) -> (-34.968, -29.0187) centre (-35.4983, -29.549) ccw projected
  arc A36 (-60.9074, -29.0187) -> (-60.377, -30.299) centre (-60.377, -29.549) ccw projected
  line L96 (-49.6877, -14.299) -> (-48.9983, -14.9883) projected
  line L97 (-78.9377, -30.299) -> (-65.4983, -30.299) projected
  arc A37 (-65.4983, -30.299) -> (-64.968, -29.0187) centre (-65.4983, -29.549) ccw projected
  arc A38 (-5.4983, -30.299) -> (-4.968, -29.0187) centre (-5.4983, -29.549) ccw projected
  arc A39 (-30.9074, -29.0187) -> (-30.377, -30.299) centre (-30.377, -29.549) ccw projected
  point P0 (0, 0)
  constraints: 2 end point
extrude "Extrusion9" add sketch "Sketch9" against normal blind 3 contours L26 L25 L24 L23 L22 L82 L18 L17 L16 L15
sketch "Sketch10" plane through (27, -12.299, 69.5623) normal (0, 1, 0) x (1, 0, 0)
  arc A0 (7.283, 13.5) -> (15.4449, 13.5) centre (11.364, 18.365) ccw projected
  line L0 (5.014, 18.365) -> (5.014, 29.865) projected
  arc A1 (9.3826, 35.898) -> (5.014, 29.865) centre (11.364, 29.865) ccw projected
  arc A2 (8.4823, 46.4158) -> (9.3826, 35.898) centre (11.364, 41.365) ccw projected
  arc A3 (17.714, 29.865) -> (13.3453, 35.898) centre (11.364, 29.865) ccw projected
  line L1 (17.714, 29.865) -> (17.714, 18.365) projected
  line L2 (70, 0) -> (0, 0) projected
  line L3 (70, 150.5) -> (70, 0) projected
  line L4 (0, 150.5) -> (70, 150.5) projected
  line L5 (0, 0) -> (0, 150.5) projected
  circle A4 centre (35, 2.1066) radius 1.45
  line L6 (7.283, 13.5) -> (6.999, 13.5) projected
  arc A5 (6.499, 14) -> (6.999, 13.5) centre (6.999, 14) ccw projected
  line L7 (6.499, 14) -> (6.499, 14.284) projected
  arc A6 (5.014, 18.365) -> (6.499, 14.284) centre (11.364, 18.365) ccw projected
  arc A7 (14.2457, 46.4158) -> (8.4823, 46.4158) centre (11.364, 47.25) ccw projected
  arc A8 (13.3453, 35.898) -> (14.2457, 46.4158) centre (11.364, 41.365) ccw projected
  arc A9 (16.229, 14.284) -> (17.714, 18.365) centre (11.364, 18.365) ccw projected
  line L8 (16.229, 14.284) -> (16.229, 14) projected
  arc A10 (15.729, 13.5) -> (16.229, 14) centre (15.729, 14) ccw projected
  line L9 (15.729, 13.5) -> (15.4449, 13.5) projected
  point P0 (-27, 69.5623)
  dimension "d93" = 2.9
  dimension "d94" = 70
  dimension "d95" = 35
  constraints: 1 centre point
  measures "d93" diameter of A4
  measures "d94" distance between parallel lines of L3 L5
  measures "d95" distance from line of L5 A4.centre
extrude "Extrusion10" cut sketch "Sketch10" against normal up to surface (5.94 mm away) contours A4
sketch "Sketch11" plane through (82, -20.739, 74.4473) normal (0, 0, 1) x (1, 0, 0)
  line L0 (-49, 2.5) -> (-49, 0) projected
  line L1 (-49, 0) -> (0, 0) projected
  line L2 (0, 2.5) -> (0, 0) projected
  line L3 (-49, 2.5) -> (0, 2.5) projected
  line L4 (0, 2.5) -> (0, 0) projected
  line L5 (0, 0) -> (2.5, 0)
  line L6 (2.5, 0) -> (2.5, 2.5)
  line L7 (2.5, 2.5) -> (0, 2.5)
  line L8 (0, 2.5) -> (0, 0)
  point P0 (-82, 20.739)
  dimension "d99" = 2.5
  constraints: 8 end point, 2 parallel, 1 horizontal, 1 perpendicular
  measures "d99" distance of L7.end L6.end
sketch "Sketch12" plane through (33, -19.739, 64.4473) normal (0, 1, 0) x (1, 0, 0)
  circle A0 centre (5.364, 13.25) radius 1.2261 projected
  line L0 (10.864, 5.75) -> (-0.136, 5.75)
  line L1 (-2.136, 7.75) -> (-2.136, 18.75)
  line L2 (-0.136, 20.75) -> (10.864, 20.75)
  line L3 (12.864, 18.75) -> (12.864, 7.75)
  line L4 (12.864, 5.75) -> (-2.136, 20.75) construction
  line L5 (-2.136, 5.75) -> (12.864, 20.75) construction
  arc A1 (-0.136, 20.75) -> (-2.136, 18.75) centre (-0.136, 18.75) ccw
  arc A2 (12.864, 18.75) -> (10.864, 20.75) centre (10.864, 18.75) ccw
  arc A3 (10.864, 5.75) -> (12.864, 7.75) centre (10.864, 7.75) ccw
  arc A4 (-2.136, 7.75) -> (-0.136, 5.75) centre (-0.136, 7.75) ccw
  line L6 (37.1916, 5.75) -> (26.1916, 5.75)
  line L7 (24.1916, 7.75) -> (24.1916, 18.75)
  line L8 (26.1916, 20.75) -> (37.1916, 20.75)
  line L9 (39.1916, 18.75) -> (39.1916, 7.75)
  line L10 (39.1916, 5.75) -> (24.1916, 20.75) construction
  line L11 (24.1916, 5.75) -> (39.1916, 20.75) construction
  arc A5 (26.1916, 20.75) -> (24.1916, 18.75) centre (26.1916, 18.75) ccw
  arc A6 (39.1916, 18.75) -> (37.1916, 20.75) centre (37.1916, 18.75) ccw
  arc A7 (37.1916, 5.75) -> (39.1916, 7.75) centre (37.1916, 7.75) ccw
  arc A8 (24.1916, 7.75) -> (26.1916, 5.75) centre (26.1916, 7.75) ccw
  point P0 (-33, 64.4473)
  dimension "d102" = 15
  dimension "d103" = 15
  dimension "d104" = 2
  dimension "d119" = 15
  dimension "d120" = 15
  dimension "d121" = 2
  constraints: 24 end point, 16 point on circle, 16 point on line, 16 tangent, 8 centre point, 6 equal radius, 4 parallel, 2 horizontal, 2 midpoint, 2 perpendicular
  measures "d102" distance of L4.end L5.end
  measures "d103" distance of L5.start L4.end
  measures "d104" radius of A1
  measures "d119" distance of L10.end L11.end
  measures "d120" distance of L11.start L10.end
  measures "d121" radius of A5
extrude "Extrusion12" cut sketch "Sketch12" against normal up to surface (2.8 mm away) contours A0 | L0 A4 L1 A1 L2 A2 L3 A3 | L6 A8 L7 A5 L8 A6 L9 A7
sketch "Sketch13" plane through (33, 0, 0) normal (-1, 0, 0) x (0, 0, 1)
  point P0 (0, 0)
sketch "Sketch14" plane through (97, 0, 0) normal (1, 0, 0) x (0, 0, -1)
  line L0 (-33.4473, -19.739) -> (-35.4473, -19.739) projected
  line L1 (-35.4473, -19.739) -> (-35.4473, -18.239) projected
  line L2 (-35.4473, -18.239) -> (-37.4473, -18.239) projected
  line L3 (-37.4473, -18.239) -> (-37.4473, -19.739) projected
  line L4 (-37.4473, -19.739) -> (-64.4473, -19.739) projected
  line L5 (-64.4473, -19.739) -> (-64.4473, -18.239) projected
  line L6 (-64.4473, -18.239) -> (-74.4473, -18.239) projected
  line L7 (-74.4473, -18.239) -> (-74.4473, -20.739) projected
  line L8 (-74.4473, -20.739) -> (-33.4473, -20.739) projected
  line L9 (-33.4473, -19.739) -> (-33.4473, -20.739) projected
  line L10 (-67.0836, -28.6297) -> (-67.0836, -25.1023) projected
  line L11 (-42.4673, -24.299) -> (-26.6973, -24.299) projected
  line L12 (-66.0057, -16.239) -> (-68.9057, -16.239) projected
  line L13 (-56.3123, -16.239) -> (-67.3123, -16.239) projected
  line L14 (-56.3123, -16.239) -> (-70.3123, -16.239) projected
  line L15 (-70.3123, -16.239) -> (-67.3123, -16.239) projected
  line L16 (-67.3123, -22.539) -> (-54.4573, -22.539) projected
  line L17 (-67.3123, -22.539) -> (-70.3123, -22.539) projected
  line L18 (-70.3123, -22.539) -> (-54.4573, -22.539) projected
  line L19 (-44.2273, -22.539) -> (-54.4573, -22.539) projected
  line L20 (-44.2273, -22.539) -> (-33.4473, -22.539) projected
  line L21 (-44.2273, -22.539) -> (-33.4473, -22.539) projected
  line L22 (-54.4573, -22.539) -> (-44.2273, -22.539) projected
  line L23 (-44.2273, -22.539) -> (-33.4473, -22.539) projected
  line L24 (-67.0836, -16.239) -> (-37.4473, -16.239)
  line L25 (-37.4473, -16.239) -> (-37.4473, -22.539)
  line L26 (-37.4473, -22.539) -> (-67.0836, -22.539)
  line L27 (-67.0836, -22.539) -> (-67.0836, -16.239)
  point P0 (0, 0)
  point P1 (-44.2273, -22.539)
  point P2 (-43.6973, -22.539)
  point P3 (-43.6973, -22.539)
  point P4 (-44.2273, -22.539)
  constraints: 8 end point, 2 parallel, 1 horizontal, 1 perpendicular, 1 point on line, 2 other
extrude "Extrusion13" cut sketch "Sketch14" against normal up to surface (10 mm away) contours L25 L20 L19 L16 L27 L8 | L8 L27 L6 L5 L4 L25 | L3 L4 L5 L6 L27 L12 L13 L24 L25
sketch "Sketch15" plane through (97, 0, 0) normal (1, 0, 0) x (0, 0, -1)
  line L0 (30.377, -30.299) -> (5.4983, -30.299) projected
  arc A0 (4.968, -29.0187) -> (5.4983, -30.299) centre (5.4983, -29.549) ccw projected
  line L1 (17.4074, -16.5793) -> (4.968, -29.0187) projected
  arc A1 (18.468, -16.5793) -> (17.4074, -16.5793) centre (17.9377, -17.1096) ccw projected
  line L2 (30.9074, -29.0187) -> (18.468, -16.5793) projected
  arc A2 (30.377, -30.299) -> (30.9074, -29.0187) centre (30.377, -29.549) ccw projected
  line L3 (79.6877, -16.1096) -> (79.6877, -29.549) projected
  arc A3 (78.9377, -30.299) -> (79.6877, -29.549) centre (78.9377, -29.549) ccw projected
  line L4 (78.9377, -30.299) -> (65.4983, -30.299) projected
  arc A4 (64.968, -29.0187) -> (65.4983, -30.299) centre (65.4983, -29.549) ccw projected
  line L5 (78.4074, -15.5793) -> (64.968, -29.0187) projected
  arc A5 (79.6877, -16.1096) -> (78.4074, -15.5793) centre (78.9377, -16.1096) ccw projected
  line L6 (-52.6092, -28.6297) -> (-67.0836, -28.6297) projected
  line L7 (-67.0836, -28.6297) -> (-67.0836, -25.1023) projected
  line L8 (-67.0836, -25.1023) -> (-56.1367, -25.1023) projected
  line L9 (-56.1367, -25.1023) -> (-52.6092, -28.6297) projected
  arc A6 (-70.3123, -31.549) -> (-69.5623, -32.299) centre (-69.5623, -31.549) ccw projected
  line L10 (-69.5623, -32.299) -> (80.9377, -32.299) projected
  arc A7 (80.9377, -32.299) -> (81.6877, -31.549) centre (80.9377, -31.549) ccw projected
  line L11 (81.6877, -31.549) -> (81.6877, -13.049) projected
  arc A8 (81.6877, -13.049) -> (80.9377, -12.299) centre (80.9377, -13.049) ccw projected
  line L12 (80.9377, -12.299) -> (-69.5623, -12.299) projected
  arc A9 (-69.5623, -12.299) -> (-70.3123, -13.049) centre (-69.5623, -13.049) ccw projected
  line L13 (-70.3123, -13.049) -> (-70.3123, -31.549) projected
  line L14 (49.6877, -14.299) -> (75.7557, -14.299) projected
  arc A10 (76.286, -15.5793) -> (75.7557, -14.299) centre (75.7557, -15.049) ccw projected
  line L15 (63.468, -28.3973) -> (76.286, -15.5793) projected
  arc A11 (62.4074, -28.3973) -> (63.468, -28.3973) centre (62.9377, -27.867) ccw projected
  line L16 (48.9983, -14.9883) -> (62.4074, -28.3973) projected
  line L17 (49.6877, -14.299) -> (48.9983, -14.9883) projected
  line L18 (60.377, -30.299) -> (35.4983, -30.299) projected
  arc A12 (34.968, -29.0187) -> (35.4983, -30.299) centre (35.4983, -29.549) ccw projected
  line L19 (47.4074, -16.5793) -> (34.968, -29.0187) projected
  arc A13 (48.468, -16.5793) -> (47.4074, -16.5793) centre (47.9377, -17.1096) ccw projected
  line L20 (60.9074, -29.0187) -> (48.468, -16.5793) projected
  arc A14 (60.377, -30.299) -> (60.9074, -29.0187) centre (60.377, -29.549) ccw projected
  line L21 (19.6877, -14.299) -> (46.1877, -14.299) projected
  line L22 (46.877, -14.9883) -> (46.1877, -14.299) projected
  line L23 (33.468, -28.3973) -> (46.877, -14.9883) projected
  arc A15 (32.4074, -28.3973) -> (33.468, -28.3973) centre (32.9377, -27.867) ccw projected
  line L24 (18.9983, -14.9883) -> (32.4074, -28.3973) projected
  line L25 (19.6877, -14.299) -> (18.9983, -14.9883) projected
  line L26 (-9.8803, -14.299) -> (16.1877, -14.299) projected
  line L27 (16.877, -14.9883) -> (16.1877, -14.299) projected
  line L28 (3.468, -28.3973) -> (16.877, -14.9883) projected
  arc A16 (2.4074, -28.3973) -> (3.468, -28.3973) centre (2.9377, -27.867) ccw projected
  line L29 (-10.4107, -15.5793) -> (2.4074, -28.3973) projected
  arc A17 (-9.8803, -14.299) -> (-10.4107, -15.5793) centre (-9.8803, -15.049) ccw projected
  line L30 (0.377, -30.299) -> (-12.9473, -30.299) projected
  arc A18 (-13.6973, -29.549) -> (-12.9473, -30.299) centre (-12.9473, -29.549) ccw projected
  line L31 (-13.6973, -29.549) -> (-13.6973, -14.414) projected
  line L32 (0.9074, -29.0187) -> (-13.6973, -14.414) projected
  arc A19 (0.377, -30.299) -> (0.9074, -29.0187) centre (0.377, -29.549) ccw projected
  line L33 (-46.0823, -16.239) -> (-37.4473, -16.239) projected
  line L34 (-37.4473, -16.239) -> (-37.4473, -22.539) projected
  line L35 (-37.4473, -22.539) -> (-44.2273, -22.539) projected
  line L36 (-44.2273, -22.539) -> (-42.4673, -24.299) projected
  line L37 (-42.4673, -24.299) -> (-26.6973, -24.299) projected
  line L38 (-26.6973, -24.299) -> (-21.6973, -19.299) projected
  line L39 (-21.6973, -19.299) -> (-21.6973, -15.299) projected
  line L40 (-21.6973, -15.299) -> (-16.6973, -15.299) projected
  line L41 (-16.6973, -15.299) -> (-16.6973, -23.299) projected
  line L42 (-16.6973, -23.299) -> (-22.1633, -28.765) projected
  line L43 (-22.1633, -28.765) -> (-48.2313, -28.765) projected
  line L44 (-48.2313, -28.765) -> (-54.4573, -22.539) projected
  line L45 (-54.4573, -22.539) -> (-67.0836, -22.539) projected
  line L46 (-67.0836, -22.539) -> (-67.0836, -16.239) projected
  line L47 (-67.0836, -16.239) -> (-56.3123, -16.239) projected
  line L48 (-56.3123, -16.239) -> (-56.3123, -15.299) projected
  line L49 (-56.3123, -15.299) -> (-46.0823, -15.299) projected
  line L50 (-46.0823, -15.299) -> (-46.0823, -16.239) projected
  line L51 (-44.2273, -22.539) -> (-42.4673, -24.299) projected
  line L52 (-42.4673, -24.299) -> (-38.0013, -28.765)
  line L53 (-26.6973, -24.299) -> (-31.1633, -28.765)
  line L54 (-48.2313, -28.765) -> (-22.1633, -28.765) projected
  point P0 (0, 0)
  constraints: 4 end point, 2 point on line, 1 collinear, 1 perpendicular
extrude "Extrusion14" add sketch "Sketch15" against normal blind 3 contours L37 L53 L43 L52